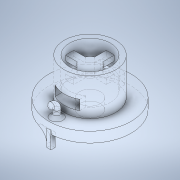
# Autodesk Inventor part: Wheel
Saved by Autodesk Inventor 2020 (Build 240168000, 168)
## iProperties
Created: 2022-03-31
Part Number: Wheel
Material: Generic
Document SubType Name: Modeling
Designer: jbwhiteh
Density: 1 g/cm^3
Appearance: Default
Mass: 16.3085 g
Surface Area: 81.5233 cm^2
Volume: 16.3085 cm^3
Author: jbwhiteh
Autodesk Inventor part; units mm, degrees
note: some values were not read from the file. Chosen so that the rebuilt part matches the saved one: second side of "Extrusion2".
sketch "Sketch1" plane through (0, 0, 0) normal (0, 1, 0) x (-1, 0, 0)
  circle A0 centre (0, 0) radius 25.4
  dimension "d0" = 50.8
  constraints: 1 centre point, 1 coincident
  measures "d0" diameter of A0
extrude "Extrusion1" add sketch "Sketch1" along normal blind 6.35
sketch "Sketch2" plane through (0, 6.35, 0) normal (0, 1, 0) x (1, 0, 0)
  circle A0 centre (0, 0) radius 25.4 projected
  point P0 (-25.4, 0)
  point P1 (0, -25.4)
  point P2 (25.4, 0)
  point P3 (0, 25.4)
  constraints: 4 point on circle
ref_plane "Work Plane1" through (0, 6.35, 25.4) normal (0, 0, 1) x (1, 0, 0)
sketch "Sketch3" plane through (0, 6.35, 25.4) normal (0, 0, 1) x (1, 0, 0)
  line L0 (1.27, -4.1248) -> (-1.27, -4.1248)
  line L1 (-1.27, -4.1248) -> (-1.27, -14.6393)
  line L2 (-1.27, -14.6393) -> (1.27, -14.6393)
  line L3 (1.27, -14.6393) -> (1.27, -4.1248)
  line L4 (25.4, 0) -> (-25.4, 0) projected
  line L5 (0, 0) -> (0, -6.35)
  dimension "d3" = 1.27
  dimension "d4" = 2.54
  constraints: 10 end point, 2 parallel, 1 horizontal, 1 midpoint, 1 perpendicular, 1 vertical
  measures "d3" distance between parallel lines of L5 L3
  measures "d4" distance of L0.start L0.end
extrude "Extrusion2" add sketch "Sketch3" against normal blind 2.54
sketch "Sketch4" plane through (0, 6.35, 0) normal (0, 1, 0) x (1, 0, 0)
  circle A0 centre (0, 0) radius 6.4452
  dimension "d9" = 12.8905
  constraints: 1 centre point, 1 coincident
  measures "d9" diameter of A0
extrude "Extrusion3" cut sketch "Sketch4" against normal blind 25.4
sketch "Sketch5" plane through (0, 6.35, 0) normal (0, 1, 0) x (1, 0, 0)
  circle A0 centre (0, 0) radius 15.875
  dimension "d12" = 31.75
  constraints: 1 centre point, 1 coincident
  measures "d12" diameter of A0
extrude "Extrusion4" add sketch "Sketch5" along normal blind 22.86
sketch "Sketch6" plane through (0, 29.21, 0) normal (0, 1, 0) x (1, 0, 0)
  circle A0 centre (0, 0) radius 12.7
  dimension "d15" = 25.4
  constraints: 1 centre point, 1 coincident
  measures "d15" diameter of A0
extrude "Extrusion5" cut sketch "Sketch6" against normal blind 19.05
sketch "Sketch7" plane through (0, 0, 0) normal (0, -1, 0) x (1, 0, 0)
  point P0 (0, 0)
sketch "Sketch8" plane through (0, 0, 0) normal (0, -1, 0) x (1, 0, 0)
  point P0 (0, 0)
sketch "Sketch9" plane through (0, 0, 0) normal (0, -1, 0) x (1, 0, 0)
  point P0 (0, 0)
sketch "Sketch10" plane through (0, 0, 0) normal (0, -1, 0) x (1, 0, 0)
  point P0 (0, 0)
ref_plane "Work Plane2" through (0, 24.13, 0) normal (0, 1, 0) x (1, 0, 0)
sketch "Sketch13" plane through (0, 24.13, 0) normal (0, 1, 0) x (1, 0, 0)
  circle A0 centre (0, 0) radius 12.7
  circle A1 centre (0, 0) radius 12.7 projected
  circle A2 centre (0, 0) radius 5.969
  line L0 (0, 12.7) -> (2.54, 12.7)
  line L1 (0, 12.7) -> (-2.54, 12.7)
  line L2 (0, -12.7) -> (2.54, -12.7)
  line L3 (2.54, -12.7) -> (2.54, 12.7)
  line L4 (0, -12.7) -> (-2.54, -12.7)
  line L5 (-2.54, -12.7) -> (-2.54, 12.7)
  line L6 (12.7, -2.54) -> (-12.7, -2.54)
  line L7 (-12.7, 0) -> (-12.7, -2.54)
  line L8 (-12.7, 0) -> (-12.7, 2.54)
  line L9 (12.7, 2.54) -> (-12.7, 2.54)
  line L10 (12.7, 0) -> (12.7, 2.54)
  line L11 (12.7, 0) -> (12.7, -2.54)
  point P0 (12.4434, -2.54)
  point P1 (5.4016, -2.54)
  point P2 (2.54, -5.4016)
  point P3 (2.54, -12.4434)
  point P4 (-5.4016, -2.54)
  point P5 (-12.4434, -2.54)
  point P6 (-2.54, -12.4434)
  point P7 (-2.54, -5.4016)
  point P8 (5.4016, 2.54)
  point P9 (12.4434, 2.54)
  point P10 (2.54, 12.4434)
  point P11 (2.54, 5.4016)
  point P12 (-12.4434, 2.54)
  point P13 (-5.4016, 2.54)
  point P14 (-2.54, 5.4016)
  point P15 (-2.54, 12.4434)
  dimension "d22" = 11.938
  dimension "d28" = 2.54
  dimension "d29" = 2.54
  dimension "d32" = 90
  constraints: 24 end point, 8 tangent, 4 horizontal, 2 centre point, 2 coincident, 2 perpendicular, 2 point on circle, 13 other
  measures "d22" diameter of A2
  measures "d28" distance of L0.start L0.end
  measures "d29" distance of L0.start L1.end
extrude "Extrusion6" add sketch "Sketch13" against normal blind 3.175 contours A0 L6 A2 L9 | L9 A2 L3 A0 | A0 L3 A2 L6 | L3 A2 L5 A0 | L9 L3 A2 | A2 L6 L3 L9 | A0 L5 A2 L3 | A2 L3 L6 | L3 L9 L5 A2 | L3 L6 L5 L9 | A2 L5 L6 L3 | L5 A2 L9 A0 | L5 L9 A2 | L5 L6 A2 L9 | A0 L6 A2 L5 | A2 L6 L5 | L9 A2 L6 A0
extrude "Extrusion7" cut sketch "Sketch13" against normal blind 3.175 contours L9 A2 L3 A0 | A0 L3 A2 L6 | L5 A2 L9 A0 | A0 L6 A2 L5
sketch "Sketch14" plane through (0, 6.35, 25.4) normal (0, 0, 1) x (1, 0, 0)
  line L0 (-12.7, 3.81) -> (12.7, 3.81) projected
  line L1 (-7.62, 9.8976) -> (7.62, 9.8976)
  line L2 (7.62, 9.8976) -> (7.62, 3.81)
  line L3 (7.62, 3.81) -> (-7.62, 3.81)
  line L4 (-7.62, 3.81) -> (-7.62, 9.8976)
  point P0 (0, -6.35)
  point P1 (-7.62, 3.81)
  dimension "d36" = 15.24
  dimension "d37" = 7.62
  constraints: 8 end point, 2 parallel, 1 horizontal, 1 perpendicular, 1 point on line
  measures "d36" distance of L1.start L1.end
  measures "d37" distance from line of point (0, -6.35) L4
extrude "Extrusion8" cut sketch "Sketch14" against normal through all
sketch "Sketch15" plane through (0, 6.35, 0) normal (0, 1, 0) x (1, 0, 0)
  circle A0 centre (0, -20.6375) radius 1.905
  circle A1 centre (0, 0) radius 15.875 projected
  circle A2 centre (0, 0) radius 25.4 projected
  dimension "d40" = 3.81
  constraints: 1 centre point
  measures "d40" diameter of A0
ref_plane "Work Plane4" through (0, 20.955, 12.4434) normal (1, 0, 0) x (0, 0, -1)
sketch "Sketch17" plane through (0, 20.955, 12.4434) normal (1, 0, 0) x (0, 0, -1)
  line L0 (-6.2891, -14.605) -> (-10.0991, -14.605) projected
  line L1 (-8.1941, -14.605) -> (-8.1941, -10.16)
  line L2 (-11.3691, -6.985) -> (-12.9566, -6.985)
  arc A0 (-8.1941, -10.16) -> (-11.3691, -6.985) centre (-11.3691, -10.16) ccw
  point P0 (12.4434, -20.955)
  point P1 (-8.1941, -6.985)
  dimension "d46" = 7.62
  dimension "d47" = 4.7625
  dimension "d48" = 3.175
  constraints: 4 end point, 2 point on circle, 2 point on line, 2 tangent, 1 centre point, 1 horizontal, 1 midpoint, 1 vertical
  measures "d46" distance of L1.start point (-8.194, -6.985)
  measures "d47" distance of point (-8.194, -6.985) L2.end
  measures "d48" radius of A0
sweep "Sweep1" add profiles "Sketch15" path "Sketch17" path curves L1 A0 L2 contours A0
fillet "Fillet1" radius 1.905 1 edges at (-1.905, 13.97, 25.4)
fillet "Fillet2" radius 1.905 1 edges at (-1.905, 6.35, 20.6375)
fillet "Fillet3" radius 6.35 1 edges at (-1.27, 0, 24.1141)
body "Solid1"
